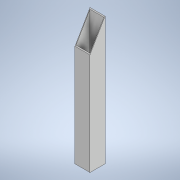
# Autodesk Inventor part: Деталь8
Saved by Autodesk Inventor 2022.4 (Build 264492010, 492A)
## iProperties
Created: 2023-02-20
Part Number: Деталь8
Material: Типовые
Document SubType Name: Modeling
Designer: artyo
Density: 1 g/cm^3
Appearance: По умолчанию
Author: artyo
Autodesk Inventor part; units mm, degrees
ref_plane "YZ Plane" through (0, 0, 0) normal (1, 0, 0) x (0, 1, 0)
ref_plane "XZ Plane" through (0, 0, 0) normal (0, 1, 0) x (-1, 0, 0)
ref_plane "XY Plane" through (0, 0, 0) normal (0, 0, 1) x (1, 0, 0)
sketch "Эскиз1" plane through (0, 0, 0) normal (0, 1, 0) x (-1, 0, 0)
  line L0 (-10, -10) -> (10, -10)
  line L1 (10, -10) -> (10, 10)
  line L2 (10, 10) -> (-10, 10)
  line L3 (-10, 10) -> (-10, -10)
  line L4 (-10, -10) -> (10, 10) construction
  line L5 (10, -10) -> (-10, 10) construction
  line L6 (-9.25, -9.25) -> (9.25, -9.25)
  line L7 (9.25, -9.25) -> (9.25, 9.25)
  line L8 (9.25, 9.25) -> (-9.25, 9.25)
  line L9 (-9.25, 9.25) -> (-9.25, -9.25)
  line L10 (-9.25, -9.25) -> (9.25, 9.25) construction
  line L11 (9.25, -9.25) -> (-9.25, 9.25) construction
  point P0 (0, 0)
  dimension "d0" = 20
  dimension "d1" = 20
  dimension "d2" = 18.5
  dimension "d3" = 18.5
  constraints: 24 end point, 4 midpoint, 4 parallel, 2 horizontal, 2 perpendicular
  measures "d0" distance of L2.end L1.end
  measures "d1" distance of L1.end L0.end
  measures "d2" distance of L8.end L7.end
  measures "d3" distance of L7.end L6.end
extrude "Выдавливание1" add sketch "Эскиз1" along normal blind 50 and the other way blind 120
sketch "Эскиз2" plane through (10, -120, 10) normal (1, 0, 0) x (0, 0, -1)
  line L0 (20, 0) -> (20, 170) projected
  line L1 (20, 170) -> (0, 135.359)
  line L2 (0, 0) -> (0, 170) projected
  line L3 (20, 170) -> (60, 170) construction
  line L4 (20, 170) -> (0, 170) projected
  line L5 (0, 135.359) -> (0, 170)
  line L6 (0, 170) -> (20, 170)
  point P0 (10, 120)
  dimension "d6" = 120
  constraints: 8 end point, 1 collinear, 1 equal length, 1 horizontal, 1 point on line, 1 vertical
  measures "d6" angle of L1 L3
extrude "Выдавливание2" cut sketch "Эскиз2" against normal blind 50
